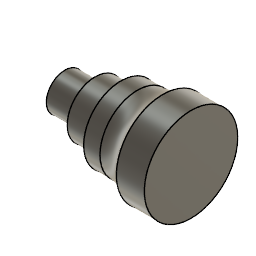
TURNING (Autodesk Fusion 360 design; units mm, degrees)
part number: 2026-06-20-14-05-09-894
Autodesk Fusion 360 part; units mm, degrees
sketch "Sketch1" plane through (0, 0, 0) normal (0, 0, 1) x (1, 0, 0)
  line L0 (0, 0) -> (-27, 0)
  line L1 (-27, 0) -> (-27, 4)
  line L2 (-27, 4) -> (-20.5209, 4)
  line L3 (-20.5209, 4) -> (-20.5209, 6)
  line L4 (-20.5209, 6) -> (-16, 6)
  line L5 (-16, 6) -> (-15, 8)
  line L6 (-15, 8) -> (-11.4968, 8)
  arc A0 (-11.4968, 8) -> (-6, 10) centre (-11.4968, 16.5538) ccw
  line L7 (-6, 10) -> (0, 10)
  line L8 (0, 10) -> (0, 0)
  dimension "d1" = 4
  dimension "d2" = 27
  constraint coincident L0.start L8.end
  constraint horizontal L0
  constraint perpendicular L0 L1
  constraint perpendicular L1 L2
  constraint perpendicular L2 L3
  constraint perpendicular L3 L4
  constraint perpendicular L3 L6
  constraint tangent L6 A0
  constraint horizontal L7
  constraint perpendicular L7 L8
  measures "d1" distance of L0.end L1.end
  measures "d2" distance of L0.start L0.end
revolve "Revolve1" add sketch "Sketch1" angle 360 about axis through (0, 0, 0) along (-1, 0, 0)
